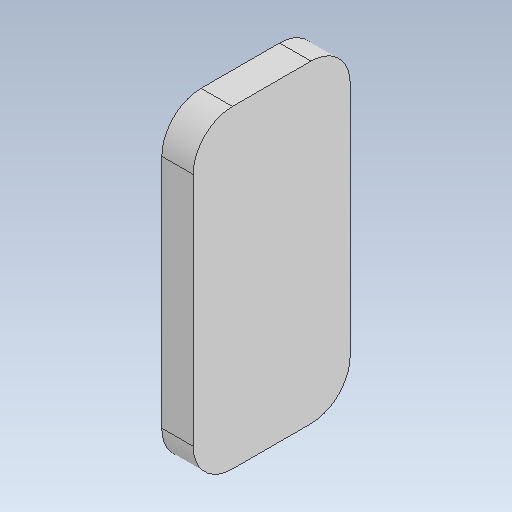
# Autodesk Inventor part: Domino
Saved by Autodesk Inventor 2021 (Build 250183000, 183)
## iProperties
Created: 2021-02-17
Part Number: Domino
Material: Generic
Document SubType Name: Modeling
Designer: david
Density: 1 g/cm^3
Appearance: Default
Author: david
Autodesk Inventor part; units mm, degrees
ref_plane "YZ Plane" through (0, 0, 0) normal (1, 0, 0) x (0, 1, 0)
ref_plane "XZ Plane" through (0, 0, 0) normal (0, 1, 0) x (-1, 0, 0)
ref_plane "XY Plane" through (0, 0, 0) normal (0, 0, 1) x (1, 0, 0)
sketch "Sketch1" plane through (0, 0, 0) normal (1, 0, 0) x (0, 1, 0)
  line L0 (3.175, -12.7) -> (22.225, -12.7)
  line L1 (25.4, -15.875) -> (25.4, -22.225)
  line L2 (22.225, -25.4) -> (3.175, -25.4)
  line L3 (0, -22.225) -> (0, -15.875)
  arc A0 (25.4, -15.875) -> (22.225, -12.7) centre (22.225, -15.875) ccw
  arc A1 (22.225, -25.4) -> (25.4, -22.225) centre (22.225, -22.225) ccw
  arc A2 (0, -22.225) -> (3.175, -25.4) centre (3.175, -22.225) ccw
  arc A3 (3.175, -12.7) -> (0, -15.875) centre (3.175, -15.875) ccw
  point P0 (0, 0)
  point P1 (0, -12.7)
  point P2 (25.4, -25.4)
  point P3 (0, -25.4)
  dimension "d0" = 25.4
  dimension "d1" = 12.7
  dimension "d2" = 3.175
  constraints: 8 end point, 8 point on circle, 8 tangent, 6 point on line, 4 centre point, 3 equal radius, 2 parallel, 1 horizontal, 1 perpendicular
  measures "d0" distance of point (25.4, -25.4) point (0, -25.4)
  measures "d1" distance of point (0, -25.4) point (0, -12.7)
  measures "d2" radius of A0
extrude "Extrusion1" add sketch "Sketch1" along normal blind 2.54
body "Solid1"
